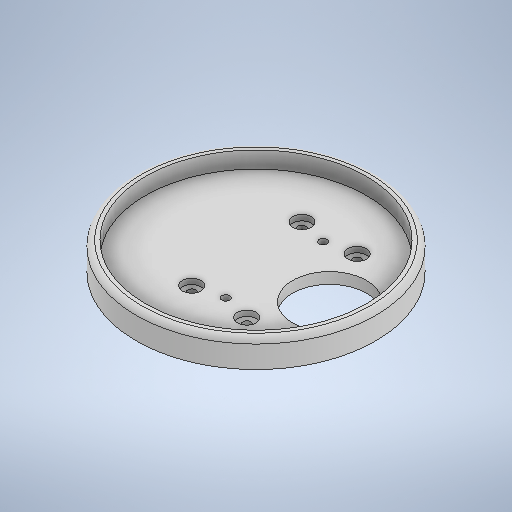
# Autodesk Inventor part: siren
Saved by Autodesk Inventor 2026.1 (Build 301233000, 233)
## iProperties
Created: 2026-05-25
Part Number: siren
Material: Generic
Document SubType Name: Modeling
Designer: chris
Density: 1 g/cm^3
Appearance: Default
Author: chris
Autodesk Inventor part; units mm, degrees
ref_plane "YZ Plane" through (0, 0, 0) normal (1, 0, 0) x (0, 1, 0)
ref_plane "XZ Plane" through (0, 0, 0) normal (0, 1, 0) x (-1, 0, 0)
ref_plane "XY Plane" through (0, 0, 0) normal (0, 0, 1) x (1, 0, 0)
sketch "Sketch1" plane through (0, 0, 0) normal (0, 1, 0) x (-1, 0, 0)
  circle A0 centre (0, 0) radius 60
  circle A1 centre (0, 0) radius 65
  dimension "d0" = 120
  dimension "d1" = 130
  constraints: 2 centre point, 2 coincident
  measures "d0" diameter of A0
  measures "d1" diameter of A1
extrude "Extrusion1" add sketch "Sketch1" along normal blind 15
sketch "Sketch4" plane through (0, 0, 0) normal (0, -1, 0) x (1, 0, 0)
  circle A0 centre (0, 0) radius 60 projected
  circle A1 centre (0, 0) radius 60
  constraints: 1 centre point, 1 coincident, 1 concentric
extrude "Extrusion4" add sketch "Sketch4" against normal blind 6
sketch "Sketch5" plane through (0, 6, 0) normal (0, 1, 0) x (1, 0, 0)
  circle A0 centre (25, -30) radius 2.1
  circle A1 centre (25, 30) radius 2.1
  circle A2 centre (-5, 30) radius 2.1
  circle A3 centre (-5, -30) radius 2.1
  point P0 (0, 0)
  dimension "d19" = 4.2
  dimension "d20" = 4.2
  dimension "d21" = 4.2
  dimension "d22" = 4.2
  dimension "d23" = 30
  dimension "d24" = 30
  dimension "d25" = 5
  dimension "d26" = 25
  constraints: 4 centre point, 2 horizontal alignment, 2 vertical alignment
  measures "d19" diameter of A0
  measures "d20" diameter of A1
  measures "d21" diameter of A2
  measures "d22" diameter of A3
  measures "d23" vertical distance of A3.centre point (0, 0)
  measures "d24" vertical distance of A2.centre point (0, 0)
  measures "d25" horizontal distance of A2.centre point (0, 0)
  measures "d26" horizontal distance of point (0, 0) A1.centre
extrude "Extrusion5" cut sketch "Sketch5" against normal blind 6
sketch "Sketch6" plane through (0, 6, 0) normal (0, 1, 0) x (1, 0, 0)
  circle A0 centre (10, -26.5) radius 2.1
  circle A1 centre (10, 26.5) radius 2.1
  point P0 (0, 0)
  dimension "d29" = 4.2
  dimension "d30" = 4.2
  dimension "d51" = 26.5
  dimension "d52" = 26.5
  dimension "d54" = 10
  constraints: 2 centre point, 1 vertical alignment
  measures "d29" diameter of A0
  measures "d30" diameter of A1
  measures "d51" vertical distance of point (0, 0) A0.centre
  measures "d52" vertical distance of A1.centre point (0, 0)
  measures "d54" horizontal distance of A0.centre point (0, 0)
extrude "Extrusion6" cut sketch "Sketch6" against normal blind 6
sketch "Sketch7" plane through (0, 6, 0) normal (0, 1, 0) x (1, 0, 0)
  circle A0 centre (40, 0) radius 20
  point P0 (0, 0)
  dimension "d35" = 40
  dimension "d39" = 40
  constraints: 1 centre point, 1 horizontal alignment
  measures "d35" diameter of A0
  measures "d39" distance of A0.centre point (0, 0)
extrude "Extrusion7" cut sketch "Sketch7" against normal blind 6
sketch "Sketch8" plane through (0, 6, 0) normal (0, 1, 0) x (1, 0, 0)
  circle A0 centre (0, 0) radius 60 projected
  circle A1 centre (40, 0) radius 20 projected
  circle A2 centre (25, 30) radius 2.1 projected
  circle A3 centre (-5, 30) radius 2.1 projected
  circle A4 centre (25, -30) radius 2.1 projected
  circle A5 centre (-5, -30) radius 2.1 projected
  circle A6 centre (10, 26.5) radius 2.1 projected
  circle A7 centre (10, -26.5) radius 2.1 projected
  circle A8 centre (25, 30) radius 5
  circle A9 centre (25, -30) radius 5
  circle A10 centre (-5, 30) radius 5
  circle A11 centre (-5, -30) radius 5
  point P0 (60, 0)
  dimension "d40" = 10
  dimension "d41" = 10
  dimension "d42" = 10
  dimension "d43" = 10
  constraints: 4 centre point, 4 coincident, 2 horizontal alignment
  measures "d40" diameter of A8
  measures "d41" diameter of A9
  measures "d42" diameter of A10
  measures "d43" diameter of A11
extrude "Extrusion8" cut sketch "Sketch8" against normal blind 3 contours A8 | A9 | A10 | A11
sketch "Sketch9" plane through (0, 0, 0) normal (0, -1, 0) x (1, 0, 0)
  circle A0 centre (40, 0) radius 20 projected
  circle A1 centre (10, 26.5) radius 2.1 projected
  circle A2 centre (10, -26.5) radius 2.1 projected
  circle A3 centre (-5, 30) radius 2.1 projected
  circle A4 centre (25, 30) radius 2.1 projected
  circle A5 centre (-5, -30) radius 2.1 projected
  circle A6 centre (25, -30) radius 2.1 projected
  circle A7 centre (0, 0) radius 65 projected
  circle A8 centre (10, 26.5) radius 5
  circle A9 centre (10, -26.5) radius 5
  dimension "d46" = 10
  dimension "d47" = 10
  constraints: 2 centre point, 2 coincident
  measures "d46" diameter of A8
  measures "d47" diameter of A9
extrude "Extrusion9" cut sketch "Sketch9" against normal blind 3 contours A8 | A9
fillet "Fillet1" radius 3 1 edges at (65, 15, 0)
body "Solid1"
